Autodesk Fusion 360 part; units mm, degrees
(part 2 of 2)
  constraint concentric A9 A250
  constraint tangent L227 A238
  constraint tangent A247 L238
  constraint tangent L229 A240
  constraint tangent L230 A241
  constraint tangent L231 A242
  constraint tangent A246 L237
  constraint tangent L233 A244
  constraint tangent L235 A245
  constraint tangent L237 A247
  constraint tangent L239 A248
  constraint tangent L241 A249
  constraint tangent A239 L243
  constraint tangent A238 L244
  constraint tangent A243 L245
  constraint tangent A242 L247
  constraint tangent L228 A251
  constraint tangent L229 A251
  constraint tangent L243 A252
  constraint tangent L244 A252
  constraint tangent L226 A253
  constraint tangent L227 A253
  constraint tangent L240 A254
  constraint tangent L241 A254
  constraint tangent L238 A255
  constraint tangent L239 A255
  constraint tangent L234 A256
  constraint tangent L235 A256
  constraint tangent L232 A257
  constraint tangent L233 A257
  constraint tangent L245 A258
  constraint tangent L246 A258
  constraint tangent L246 A259
  constraint tangent L247 A259
  constraint tangent L248 A260
  constraint tangent L248 A261
  constraint coincident L220 L249.start
  constraint perpendicular L220 L249
  constraint perpendicular L249 L250
  constraint tangent L250 A262
  constraint coincident L249.start A262.end
  constraint tangent L250 A263
  constraint coincident L220 L251.start
  constraint coincident L237 L251.end
  constraint perpendicular L237 L251
  constraint coincident L221 L252.start
  constraint coincident L238 L252.end
  constraint perpendicular L238 L252
  measures "d1" diameter of A0
  measures "d2" diameter of A1
  measures "d3" diameter of A2
  measures "d4" diameter of A3
  measures "d5" diameter of A4
  measures "d9" diameter of A111
  measures "d12" diameter of A112
  measures "d367" diameter of A202
  measures "d368" diameter of A203
  measures "d369" diameter of A204
  measures "d370" diameter of A205
extrude "Extrude1" add sketch "mriya-classic-fdm-301645" along normal blind 12 contours L204 A216 L205 A217 L206 A218 L207 A219 L208 A220 L209 A221 L210 A222 L211 A223 L212 A224 L213 A225 L214 A226 L215 A227 L216 A228 L217 A229 L218 A230 L219 A231 L220 L221 A233 L222 A234 L223 A235 L224 A236 L225 A237 L226 L227 A238 A239 L228 L229 A240 L230 A241 L231 A242 A243 L232 L233 A244 L234 L235 A245 L236 A246 L237 L238 L239 A248 L240 L241 A249 L242 A250 L243 L244 L245 L246 L247 A251 A252 A253 A254 A255 A256 A257 A258 A259 L251 L252 makes body 1
extrude "Extrude2" add sketch "mriya-classic-fdm-301645" along normal blind 18.5 contours L220 A232 L221 L237 A247 L238 L251 L252 bodies 1
extrude "Extrude3" add sketch "mriya-classic-fdm-301645" along normal blind 5.2 contours A114 | A115 | A116 | A117 | L204 A216 L205 A217 L206 A218 L207 A219 L208 A220 L209 A221 L210 A222 L211 A223 L212 A224 L213 A225 L214 A226 L215 A227 L216 A228 L217 A229 L218 A230 L219 A231 L220 A232 L221 A233 L222 A234 L223 A235 L224 A236 L225 A237 L248 A260 A261 L250 A262 A263 | L221 L248 A260 A261 | L220 L250 A262 A263 bodies 1
extrude "Extrude13" add sketch "mriya-classic-fdm-301645" along normal blind 3.2 contours A2 | L108 L109 A118 A119 A120 L181 L182 A206 | A121 L110 A122 L111 A123 L176 L177 A207 | A124 L112 A125 L113 A126 L114 A127 L115 | A128 L116 A129 L117 A130 L118 A131 L119 | A132 L120 A133 A134 L121 L183 L184 L185 A194 A195 | A135 L122 A136 A137 L123 L178 L179 L180 A196 A197 | A138 L124 A139 L125 A140 L126 A141 L127 | A142 L128 A143 L129 A144 L130 A145 L131 | A146 L132 A147 L133 A148 L134 A149 L135 | A150 L136 A151 L137 A152 L138 A153 L139 | A154 L140 A155 L141 A156 L142 A157 L143 | A158 L144 A159 L145 A160 L146 A161 L147 | A162 L148 A163 L149 A164 L150 A165 L151 | A166 L152 A167 L153 A168 L188 L189 L190 A198 A199 | A169 L154 A170 L155 A171 L156 A172 L157 | A173 L158 A174 L159 A175 L193 L194 L195 A200 A201 | A176 L160 A177 L161 A178 L162 A179 L163 | A180 A181 L164 A182 L165 L191 L192 A209 | A183 L166 A184 L167 A185 L168 A186 L169 | A187 A188 L170 A189 L171 L186 L187 A208 | A190 L172 A191 L173 A192 L174 A193 L175 bodies 1
extrude "Extrude14" add sketch "mriya-classic-fdm-301645" along normal blind 3.2 contours A0 | A1 | A3 | A4 bodies 1
extrude "Extrude6" add sketch "mriya-classic-fdm-301645" along normal blind 1.2 from surface at 15.6 contours L221 L248 A260 A261 bodies 1
extrude "Extrude12" add sketch "mriya-classic-fdm-301645" along normal blind 1.2 from surface at 9 contours L220 L250 A262 A263 bodies 1
extrude "Extrude21" add sketch "mriya-classic-fdm-301645" along normal blind 2.7 contours L196 L201 L202 A212 A213 L203 | L196 L197 L200 L202 A214 A215 bodies 1
extrude "Extrude19" add sketch "mriya-classic-fdm-301645" along normal blind 1.2 contours L196 L200 L202 L203 bodies 1
chamfer "Chamfer26" distance 0.7 angle 45 2 edges at (-16.35, 78.2132, 15.6) (-6.88, 9.5932, 9) measured on face at (-25.3572, 78.2132, 7.4667) measured on face at (-6.88, 57.4599, 11.9) on bodies 1
sketch "power switch" plane through (-4.28, 0, 0) normal (1, 0, 0) x (0, 1, 0)
  line L0 (24.0932, 6) -> (24.0932, 10.7)
  line L1 (37.2932, 5.6) -> (24.4932, 5.6)
  arc A0 (37.6932, 10.7) -> (37.2932, 11.1) centre (37.2932, 10.7) ccw
  line L2 (36.0932, 9.8) -> (36.0932, 6.9)
  line L3 (25.6932, 9.8) -> (36.0932, 9.8)
  line L4 (36.0932, 6.9) -> (25.6932, 6.9)
  line L5 (25.6932, 6.9) -> (25.6932, 9.8)
  line L6 (24.4932, 11.1) -> (37.2932, 11.1)
  arc A1 (24.0932, 6) -> (24.4932, 5.6) centre (24.4932, 6) ccw
  arc A2 (37.2932, 5.6) -> (37.6932, 6) centre (37.2932, 6) ccw
  line L7 (37.6932, 10.7) -> (37.6932, 6)
  arc A3 (24.4932, 11.1) -> (24.0932, 10.7) centre (24.4932, 10.7) ccw
  line L8 (1.9932, 0) -> (76.4932, 0)
  line L9 (76.4932, 0) -> (76.4932, 18.5)
  line L10 (76.4932, 18.5) -> (19.3932, 18.5)
  line L11 (19.3932, 18.5) -> (19.3932, 12)
  line L12 (19.3932, 12) -> (1.9932, 12)
  line L13 (1.9932, 12) -> (1.9932, 0)
  constraint perpendicular L4 L5
  constraint vertical L5
  constraint perpendicular L3 L5
  constraint vertical L2
  constraint tangent A0 L6
  constraint tangent A0 L7
  constraint tangent A2 L7
  constraint tangent L1 A2
  constraint tangent L1 A1
  constraint tangent L0 A1
  constraint tangent L0 A3
  constraint tangent L6 A3
extrude "Extrude8" cut sketch "power switch" against normal blind 2.6 contours L2 L3 L4 L5 bodies 1
extrude "Extrude9" cut sketch "power switch" against normal blind 1.2 contours L0 L1 A0 L6 A1 A2 L7 A3 bodies 1
chamfer "Chamfer27" distance 1.43 angle 40 8 edges at (-4.28, 30.8932, 5.6) (-4.28, 24.2104, 5.7172) (-4.28, 24.0932, 8.35) (-4.28, 24.2104, 10.9828) (-4.28, 30.8932, 11.1) (-4.28, 37.576, 10.9828) (-4.28, 37.6932, 8.35) (-4.28, 37.576, 5.7172) measured on face at (-4.28, 63.5599, 9.7333) measured on face at (-4.28, 63.5599, 9.7333) measured on face at (-4.28, 63.5599, 9.7333) measured on face at (-4.28, 63.5599, 9.7333) measured on face at (-4.28, 63.5599, 9.7333) measured on face at (-4.28, 63.5599, 9.7333) measured on face at (-4.28, 63.5599, 9.7333) measured on face at (-4.28, 63.5599, 9.7333) on bodies 1
sketch "usb-c" plane through (0, 80.8132, 0) normal (0, 1, 0) x (-1, 0, 0)
  line L0 (19.8002, 10.3) -> (13.0002, 10.3)
  line L1 (21.8002, 14.5) -> (21.8002, 9.7)
  line L2 (21.0002, 12.7) -> (21.0002, 11.5)
  arc A0 (11.4002, 14.9) -> (11.0002, 14.5) centre (11.4002, 14.5) ccw
  arc A1 (21.4002, 9.3) -> (21.8002, 9.7) centre (21.4002, 9.7) ccw
  line L3 (11.8003, 11.5) -> (11.8003, 12.7)
  line L4 (21.4002, 9.3) -> (11.4002, 9.3)
  line L5 (11.4002, 14.9) -> (21.4002, 14.9)
  line L6 (13.0002, 13.9) -> (19.8002, 13.9)
  arc A2 (21.8002, 14.5) -> (21.4002, 14.9) centre (21.4002, 14.5) ccw
  arc A3 (11.0002, 9.7) -> (11.4002, 9.3) centre (11.4002, 9.7) ccw
  line L7 (11.0002, 9.7) -> (11.0002, 14.5)
  line L8 (8.6, 0) -> (41.0177, 0)
  line L9 (41.0177, 0) -> (41.0177, 12)
  line L10 (41.0177, 12) -> (25.7, 12)
  line L11 (25.7, 12) -> (25.7, 18.5)
  line L12 (25.7, 18.5) -> (8.6, 18.5)
  line L13 (8.6, 18.5) -> (8.6, 0)
  arc A4 (13.0002, 13.9) -> (11.8003, 12.7) centre (13.0002, 12.7) ccw
  arc A5 (11.8003, 11.5) -> (13.0002, 10.3) centre (13.0002, 11.5) ccw
  arc A6 (21.0002, 12.7) -> (19.8002, 13.9) centre (19.8002, 12.7) ccw
  arc A7 (19.8002, 10.3) -> (21.0002, 11.5) centre (19.8002, 11.5) ccw
  constraint perpendicular L1 L5
  constraint perpendicular L4 L7
  constraint horizontal L4
  constraint perpendicular L1 L4
  constraint tangent A0 L5
  constraint tangent A0 L7
  constraint tangent L5 A2
  constraint tangent L1 A2
  constraint tangent A3 L7
  constraint tangent L4 A3
  constraint tangent A1 L4
  constraint tangent L1 A1
  constraint tangent L3 A4
  constraint tangent L6 A4
  constraint tangent L0 A5
  constraint tangent L3 A5
  constraint tangent L2 A6
  constraint tangent L6 A6
  constraint tangent L0 A7
  constraint tangent L2 A7
extrude "Extrude17" cut sketch "usb-c" against normal blind 2.6 contours L0 L2 L3 L6 A4 A5 A6 A7 bodies 1
extrude "Extrude18" cut sketch "usb-c" against normal blind 1.2 contours L1 A0 A1 L4 L5 A2 A3 L7 bodies 1
chamfer "Chamfer28" distance 1.2 angle 45 8 edges at (-16.4003, 80.8132, 9.3) (-11.1174, 80.8132, 9.4172) (-11.0003, 80.8132, 12.1) (-11.1174, 80.8132, 14.7828) (-16.4003, 80.8132, 14.9) (-21.6831, 80.8132, 14.7828) (-21.8003, 80.8132, 12.1) (-21.6831, 80.8132, 9.4172) on bodies 1
chamfer "Chamfer25" distance 0.9 angle 45 6 edges at (-11.1722, 22.9091, 0) (-23.6722, 22.9091, 0) (-45.9722, 22.9591, 0) (-45.9722, 60.9591, 0) (-121.9722, 53.9591, 0) (-121.9722, 34.9591, 0) on bodies 1
chamfer "Chamfer29" distance 1.2 angle 45 87 edges at (-33.3589, 80.8132, 12) (-41.4004, 80.8893, 12) (-42.0225, 81.4038, 12) (-43.8839, 82.7463, 12) (-51.773, 83.1132, 12) (-58.2004, 83.1893, 12) (-59.9225, 84.8038, 12) (-62.8839, 87.2463, 12) (-73.4, 87.6132, 12) (-83.9161, 87.2463, 12) (-86.3775, 85.3038, 12) (-87.5996, 84.1893, 12) (-94.5269, 84.1132, 12) (-102.9161, 83.7463, 12) (-107.4811, 79.7002, 12) (-111.1311, 76.2654, 12) (-115.9841, 76.1132, 12) (-121.9161, 75.7463, 12) (-123.7775, 74.4038, 12) (-124.3996, 73.8893, 12) (-131.4411, 73.8132, 12) (-141.1547, 72.5479, 12) (-142.42, 42.8932, 12) (-141.1547, 13.2385, 12) (-120.6213, 11.9732, 12) (-100.9154, 12.4162, 12) (-96.1725, 16.5326, 12) (-92.6689, 19.821, 12) (-84.6, 19.9732, 12) (-75.7843, 19.5642, 12) (-70.8069, 11.5856, 12) (-65.1622, 2.9302, 12) (-55.7575, 2.2732, 12) (-48.3996, 2.1971, 12) (-47.7775, 1.6826, 12) (-45.9161, 0.3401, 12) (-36.927, -0.0268, 12) (-29.3996, -0.1029, 12) (-28.7775, -0.6174, 12) (-26.9161, -1.9599, 12) (-16.8358, -2.3268, 12) (-5.5453, -1.0615, 12) (-4.28, 10.6932, 12) (-24.8089, 80.8132, 0) (-5.5453, 79.5479, 0) (-4.28, 39.2432, 0) (-5.5453, -1.0615, 0) (-16.8358, -2.3268, 0) (-26.9161, -1.9599, 0) (-28.7775, -0.6174, 0) (-29.3996, -0.1029, 0) (-36.927, -0.0268, 0) (-45.9161, 0.3401, 0) (-47.7775, 1.6826, 0) (-48.3996, 2.1971, 0) (-55.7575, 2.2732, 0) (-65.1622, 2.9302, 0) (-70.8069, 11.5856, 0) (-75.7843, 19.5642, 0) (-84.6, 19.9732, 0) (-92.6689, 19.821, 0) (-96.1725, 16.5326, 0) (-100.9154, 12.4162, 0) (-120.6213, 11.9732, 0) (-141.1547, 13.2385, 0) (-142.42, 42.8932, 0) (-141.1547, 72.5479, 0) (-131.4411, 73.8132, 0) (-124.3996, 73.8893, 0) (-123.7775, 74.4038, 0) (-121.9161, 75.7463, 0) (-115.9841, 76.1132, 0) (-111.1311, 76.2654, 0) (-107.4811, 79.7002, 0) (-102.9161, 83.7463, 0) (-94.5269, 84.1132, 0) (-87.5996, 84.1893, 0) (-86.3775, 85.3038, 0) (-83.9161, 87.2463, 0) (-73.4, 87.6132, 0) (-62.8839, 87.2463, 0) (-59.9225, 84.8038, 0) (-58.2004, 83.1893, 0) (-51.773, 83.1132, 0) (-43.8839, 82.7463, 0) (-42.0225, 81.4038, 0) (-41.4004, 80.8893, 0) on bodies 1
fillet "Fillet32" radius 1.2 2 edges at (-25.7, 80.8132, 14.65) (-4.28, 19.3932, 14.65) on bodies 1
chamfer "Chamfer30" distance 1.2 angle 45 7 edges at (-4.28, 48.5432, 18.5) (-5.5453, 79.5479, 18.5) (-16.55, 80.8132, 18.5) (-25.3485, 80.4617, 18.5) (-25.7, 78.9132, 18.5) (-6.18, 19.3932, 18.5) (-4.6315, 19.7447, 18.5) on bodies 1
sketch "silicone feets" plane through (0, 0, 0) normal (0, 0, -1) x (1, 0, 0)
  circle A0 centre (-11.98, -73.1132) radius 4.1
  circle A1 centre (-73.4, -79.9132) radius 4.1
  circle A2 centre (-134.72, -66.1132) radius 4.1
  circle A3 centre (-134.72, -19.6732) radius 4.1
  circle A4 centre (-61.0521, -9.9732) radius 4.1
  circle A5 centre (-11.98, -5.3732) radius 4.1
  circle A6 centre (-120.9, -53.5432) radius 2.05
  circle A7 centre (-44.9, -22.5432) radius 2.05
  circle A8 centre (-10.1, -22.4932) radius 2.05
  circle A9 centre (-22.6, -22.4932) radius 2.05
  circle A10 centre (-44.9, -60.5432) radius 2.05
  circle A11 centre (-120.9, -34.5432) radius 2.05
  line L0 (-41.0177, -79.6132) -> (-8.6, -79.6132)
  arc A12 (-8.6, -79.6132) -> (-5.48, -76.4932) centre (-8.6, -76.4932) ccw
  line L1 (-5.48, -76.4932) -> (-5.48, -1.9932)
  arc A13 (-5.48, -1.9932) -> (-8.6, 1.1268) centre (-8.6, -1.9932) ccw
  line L2 (-8.6, 1.1268) -> (-25.0716, 1.1268)
  arc A14 (-25.0716, 1.1268) -> (-27.6313, 0.0665) centre (-25.0715, -2.4933) ccw
  line L3 (-27.6313, 0.0665) -> (-28.2267, -0.5288)
  arc A15 (-29.7823, -1.1732) -> (-28.2267, -0.5288) centre (-29.7823, 1.0268) ccw
  line L4 (-29.7823, -1.1732) -> (-44.0716, -1.1732)
  arc A16 (-44.0716, -1.1732) -> (-46.6313, -2.2335) centre (-44.0715, -4.7933) ccw
  line L5 (-46.6313, -2.2335) -> (-47.2267, -2.8288)
  arc A17 (-48.7823, -3.4732) -> (-47.2267, -2.8288) centre (-48.7823, -1.2732) ccw
  line L6 (-48.7823, -3.4732) -> (-62.7328, -3.4732)
  arc A18 (-62.7328, -3.4732) -> (-65.8846, -5.3125) centre (-62.7328, -7.0932) ccw
  line L7 (-65.8846, -5.3125) -> (-73.6397, -19.0392)
  arc A19 (-77.2964, -21.1732) -> (-73.6397, -19.0392) centre (-77.2964, -16.9732) ccw
  line L8 (-77.2964, -21.1732) -> (-91.9035, -21.1732)
  arc A20 (-94.1662, -20.2359) -> (-91.9035, -21.1732) centre (-91.9035, -17.9732) ccw
  line L9 (-94.1662, -20.2359) -> (-99.8758, -14.5263)
  arc A21 (-99.8758, -14.5263) -> (-103.1426, -13.1732) centre (-103.1426, -17.7931) ccw
  line L10 (-103.1426, -13.1732) -> (-138.1, -13.1732)
  arc A22 (-138.1, -13.1732) -> (-141.22, -16.2932) centre (-138.1, -16.2932) ccw
  line L11 (-141.22, -16.2932) -> (-141.22, -69.4932)
  arc A23 (-141.22, -69.4932) -> (-138.1, -72.6132) centre (-138.1, -69.4932) ccw
  line L12 (-138.1, -72.6132) -> (-124.7823, -72.6132)
  arc A24 (-123.2267, -73.2576) -> (-124.7823, -72.6132) centre (-124.7823, -74.8132) ccw
  line L13 (-123.2267, -73.2576) -> (-122.6313, -73.8529)
  arc A25 (-122.6313, -73.8529) -> (-120.0716, -74.9132) centre (-120.0716, -71.2933) ccw
  line L14 (-120.0716, -74.9132) -> (-111.8965, -74.9132)
  arc A26 (-109.6338, -75.8505) -> (-111.8965, -74.9132) centre (-111.8965, -78.1132) ccw
  line L15 (-109.6338, -75.8505) -> (-103.6313, -81.8529)
  arc A27 (-103.6313, -81.8529) -> (-101.0716, -82.9132) centre (-101.0716, -79.2933) ccw
  line L16 (-101.0716, -82.9132) -> (-87.9823, -82.9132)
  arc A28 (-86.4267, -83.5576) -> (-87.9823, -82.9132) centre (-87.9823, -85.1132) ccw
  line L17 (-86.4267, -83.5576) -> (-84.6313, -85.3529)
  arc A29 (-84.6313, -85.3529) -> (-82.0716, -86.4132) centre (-82.0716, -82.7933) ccw
  line L18 (-82.0716, -86.4132) -> (-64.7284, -86.4132)
  arc A30 (-64.7284, -86.4132) -> (-62.1687, -85.3529) centre (-64.7285, -82.7931) ccw
  line L19 (-62.1687, -85.3529) -> (-59.3733, -82.5576)
  arc A31 (-57.8177, -81.9132) -> (-59.3733, -82.5576) centre (-57.8177, -84.1132) ccw
  line L20 (-57.8177, -81.9132) -> (-45.7284, -81.9132)
  arc A32 (-45.7284, -81.9132) -> (-43.1687, -80.8529) centre (-45.7285, -78.2931) ccw
  line L21 (-43.1687, -80.8529) -> (-42.5733, -80.2576)
  arc A33 (-41.0177, -79.6132) -> (-42.5733, -80.2576) centre (-41.0177, -81.8132) ccw
  dimension "d374" = 8.2
  dimension "d375" = 8.2
  dimension "d376" = 8.2
  dimension "d377" = 8.2
  dimension "d378" = 8.2
  dimension "d379" = 8.2
  dimension "d511" = 6.5
  dimension "d512" = 6.5
  dimension "d513" = 6.5
  dimension "d514" = 6.5
  dimension "d515" = 6.5
  dimension "d516" = 6.5
  dimension "d517" = 6.5
  dimension "d518" = 6.5
  dimension "d519" = 6.5
  dimension "d520" = 6.5
  dimension "d521" = 6.5
  measures "d374" diameter of A0
  measures "d375" diameter of A1
  measures "d376" diameter of A2
  measures "d377" diameter of A3
  measures "d378" diameter of A4
  measures "d379" diameter of A5
  measures "d511" distance of A0.centre L1
  measures "d512" distance of A0.centre L0
  measures "d513" distance of A1.centre L18
  measures "d514" distance of A2.centre L12
  measures "d515" distance of A2.centre L11
  measures "d516" distance of A3.centre L11
  measures "d517" distance of A3.centre L10
  measures "d518" distance of A4.centre L7
  measures "d519" distance of A4.centre L6
  measures "d520" distance of A5.centre L2
  measures "d521" distance of A5.centre L1
extrude "Extrude15" cut sketch "silicone feets" against normal blind 0.8 contours A0 | A1 | A2 | A3 | A4 | A5 bodies 1
fillet "Fillet31" radius 0.8 4 edges at (-7.7, 72.0932, 1.95) (-25, 72.0932, 1.95) (-25, 24.8932, 1.95) (-7.7, 24.8932, 1.95) on bodies 1
mirror "Mirror1" about plane through (0, 0, 0) normal (1, 0, 0) of bodies 1 makes body 2
named bodies: "Left", "Left (1)"
